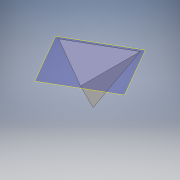
# Autodesk Inventor part: JIMSPT
Saved by Autodesk Inventor 2019 (Build 230136000, 136)
## iProperties
Created: 2019-09-15
Part Number: JIMSPT
Material: Generic
Document SubType Name: Modeling
Designer: james
Density: 1 g/cm^3
Appearance: Default
Author: james
Autodesk Inventor part; units mm, degrees
ref_plane "YZ Plane" through (0, 0, 0) normal (1, 0, 0) x (0, 1, 0)
ref_plane "XZ Plane" through (0, 0, 0) normal (0, 1, 0) x (-1, 0, 0)
sketch "Sketch1" plane through (0, 0, 0) normal (0, 1, 0) x (-1, 0, 0)
  line L0 (-6.4614, 12.7) -> (-6.4614, -12.7)
  line L1 (11.6761, 0) -> (-11.921, 0)
  line L2 (-6.4614, 12.7) -> (15.5356, 0)
  line L3 (15.5356, 0) -> (-6.4614, -12.7)
  line L4 (-6.4614, -12.7) -> (3.3823, 4.3498)
  line L5 (-6.4614, 12.7) -> (2.7414, -3.2397)
  point P0 (0, 0)
  dimension "d0" = 25.4
  dimension "d1" = 12.7
  dimension "d2" = 60
  dimension "d3" = 0
  dimension "d4" = 30
  dimension "d5" = 30
  constraints: 12 end point, 1 horizontal, 1 point on line, 1 vertical
  measures "d0" distance of L0.start L0.end
  measures "d1" vertical distance of point (0, 0) L0.start
  measures "d2" angle of L0 L2
  measures "d3" distance from line of point (0, 0) L1
  measures "d4" angle of L0 L5
  measures "d5" angle of L0 L4
ref_plane "Work Plane2" through (-15.5356, -17.9578, 0) normal (0, -1, 0) x (0.8660254, 0, -0.5)
ref_plane "Work Plane1" through (-15.5356, 0, 0) normal (0, -1, 0) x (0.8660254, 0, -0.5)
sketch "Sketch3" plane through (-15.5356, -17.9578, 0) normal (0, -1, 0) x (0.8660254, 0, -0.5)
  point P0 (13.4543, 7.7678)
  point P1 (12.6914, 7.3422)
loft "Loft1" add profiles "Sketch1" section 1 point at (-0.8734, -17.9578, 0.0128)
body "Solid2"
